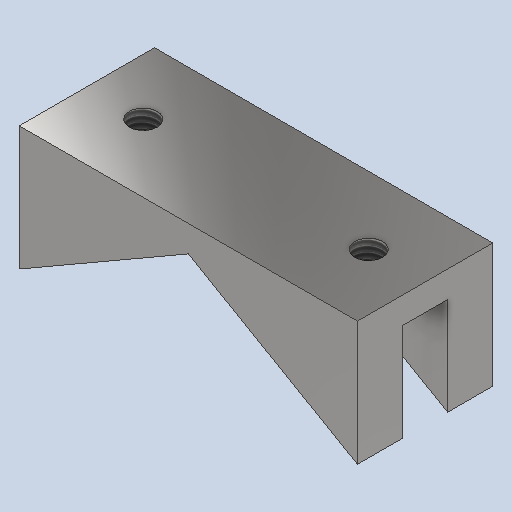
# Autodesk Inventor part: szczęka
Saved by Autodesk Inventor 2022.1 (Build 261234020, 234B)
## iProperties
Created: 2022-05-02
Part Number: szczęka
Material: Stal nierdzewna 440C
Document SubType Name: Modeling
Designer: Kacper Kaczmarski
Density: 7.75 g/cm^3
Appearance: Częściowo polerowany
Mass: 14.4102 g
Surface Area: 16.29 cm^2
Volume: 1.85937 cm^3
Author: Kacper Kaczmarski
Autodesk Inventor part; units mm, degrees
ref_plane "YZ Plane" through (0, 0, 0) normal (1, 0, 0) x (0, 1, 0)
ref_plane "XZ Plane" through (0, 0, 0) normal (0, 1, 0) x (-1, 0, 0)
ref_plane "XY Plane" through (0, 0, 0) normal (0, 0, 1) x (1, 0, 0)
sketch "Szkic1" plane through (0, 0, 0) normal (0, 0, 1) x (1, 0, 0)
  line L0 (-15.0276, 11) -> (14.9724, 11)
  line L1 (14.9724, 11) -> (14.9724, 0)
  line L2 (14.9724, 0) -> (-15.0276, 0)
  line L3 (-15.0276, 0) -> (-15.0276, 11)
  point P0 (0, 0)
  dimension "d0" = 30
  dimension "d1" = 11
  constraints: 8 end point, 2 parallel, 1 horizontal, 1 perpendicular
  measures "d0" distance of L1.end L2.end
  measures "d1" distance of L0.end L1.end
extrude "Wyciągnięcie proste1" add sketch "Szkic1" along normal blind 12
sketch "Szkic2" plane through (0, 0, 12) normal (0, 0, 1) x (1, 0, 0)
  line L0 (14.9724, 11) -> (-15.0276, 11) projected
  line L1 (-0.0276, 11) -> (0, 0)
  line L2 (-15.0276, 11) -> (-15.0276, 0) projected
  line L3 (-15.0276, 0) -> (14.9724, 0) projected
  line L4 (-15.0276, 8.66) -> (14.9724, 8.66)
  line L5 (14.9724, 0) -> (14.9724, 11) projected
  line L6 (-15.0276, 0) -> (-0.0276, 8.66)
  line L7 (-0.0276, 8.66) -> (14.9724, 0)
  line L8 (14.9724, 0) -> (-15.0276, 0)
  dimension "d4" = 8.66
  constraints: 10 end point, 2 midpoint, 2 point on line, 1 collinear, 1 horizontal
  measures "d4" distance from line of L3 L4.start
extrude "Wyciągnięcie proste2" cut sketch "Szkic2" against normal blind 12 contours L7 L3 L1 | L1 L3 L6
sketch "Szkic3" plane through (-15.0276, 11, 0) normal (-1, 0, 0) x (0, 0, 1)
  line L0 (12, -2.34) -> (0, -2.34) projected
  line L1 (0, 0) -> (12, 0) projected
  line L2 (6, 0) -> (6, -11)
  line L3 (0, -11) -> (12, -11) projected
  line L4 (8, -2.34) -> (4, -2.34)
  line L5 (4, -2.34) -> (4, -11)
  line L6 (4, -11) -> (8, -11)
  line L7 (8, -11) -> (8, -2.34)
  point P0 (4, -2.34)
  dimension "d7" = 4
  constraints: 10 end point, 2 parallel, 2 point on line, 1 horizontal, 1 midpoint, 1 perpendicular, 1 vertical, 1 other
  measures "d7" distance of L6.end L5.end
extrude "Wyciągnięcie proste3" cut sketch "Szkic3" against normal blind 30
sketch "Szkic4" plane through (-15.0276, 11, 0) normal (0, 1, 0) x (1, 0, 0)
  line L0 (0, 0) -> (0, -12) projected
  line L1 (0, -6) -> (30, -6)
  line L2 (30, 0) -> (30, -12) projected
  line L3 (30, -12) -> (0, -12) projected
  line L4 (25, -12) -> (25, 0)
  line L5 (30, 0) -> (15, 0) projected
  line L6 (15, -12) -> (15, -8) projected
  line L7 (15, 0) -> (15, -12)
  line L8 (5, -12) -> (5, 0)
  point P0 (15.0276, 0)
  point P1 (5, -6)
  point P2 (25, -6)
  dimension "d10" = 5
  constraints: 8 end point, 4 midpoint, 2 symmetric about line, 1 perpendicular, 1 point on line, 1 vertical
  measures "d10" distance between parallel lines of L2 L4
hole "Otwór1" at (-10.0276, 11, 6) at (9.9724, 11, 6) direction (0, -1, 0) diameter 2.459 depth 8.8 tip angle 118 thread size "M3x0.5" class "6H" standard "ISO Metric profile"
